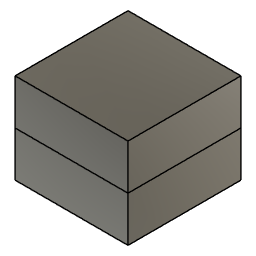
day19-parametric_modeling (Autodesk Fusion 360 design; units mm, degrees)
part number: 2025-06-29-20-21-11-885
part number: 2025-06-29-20-23-21-177
part number: 2025-06-29-20-27-52-331
Autodesk Fusion 360 part; units mm, degrees
sketch "box-width" plane through (0, 0, 0) normal (0, 0, 1) x (1, 0, 0) in component "box_bottom"
  line L0 (0, 0) -> (50, 0)
  line L1 (50, 0) -> (50, 50)
  line L2 (50, 50) -> (0, 50)
  line L3 (0, 50) -> (0, 0)
  dimension "d3" = 50
  dimension "d4" = 50
  constraint horizontal L0
  constraint vertical L1
  constraint horizontal L2
  constraint vertical L3
  constraint coincident L0.start L3.end
  measures "d3" distance of L0.start L0.end
  measures "d4" distance of L0.start L2.end
extrude "Extrude1" add sketch "box-width" along normal blind 20 makes body 1 in component "box_bottom"
shell "Shell1" thickness 2 removed faces 1 at (16.6667, 33.3333, 20) on bodies 1 in component "box_bottom"
sketch "box-width (2)" plane through (0, 0, 0) normal (0, 0, 1) x (1, 0, 0) in component "box_top"
  line L0 (0, 0) -> (50, 0)
  line L1 (50, 0) -> (50, 50)
  line L2 (50, 50) -> (0, 50)
  line L3 (0, 50) -> (0, 0)
  dimension "d3_1" = 50
  dimension "d4_1" = 50
  constraint horizontal L0
  constraint vertical L1
  constraint horizontal L2
  constraint vertical L3
  constraint coincident L0.start L3.end
  measures "d3_1" distance of L0.start L0.end
  measures "d4_1" distance of L0.start L2.end
extrude "Extrude1'" add sketch "box-width (2)" along normal blind 20 separate body makes body 2 in component "box_top"
shell "Shell1'" thickness 2 removed faces 1 at (16.6667, 33.3333, 20) on bodies 2 in component "box_top"
component "box_bottom" placed x (1, 0, 0) y (0, 1, 0) z (0, 0, 1) at (0, 0, 0)
component "box_top" placed x (-1, 0, 0) y (0, 1, 0) z (0, 0, -1) at (50, 0, 40)
equation "box_width = 50 mm"
equation "box_height = 40 mm"
equation "d3 = box_width"
equation "d4 = box_width"
equation "d5 = box_height / 2"
equation "wall_thickness = 2 mm"
equation "d3_1 = box_width"
equation "d4_1 = box_width"
equation "d5_1 = box_height / 2"
equation "wall_thickness_1 = 2 mm"
